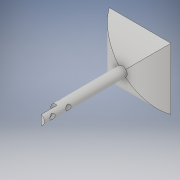
# Autodesk Inventor part: thumper-bumper-plunger
Saved by Autodesk Inventor 2017 (Build 210142000, 142)
## iProperties
Created: 2017-02-27
Part Number: thumper-bumper-plunger
Material: Generic
Document SubType Name: Modeling
Designer: John
Density: 1 g/cm^3
Appearance: Default
Author: John
Autodesk Inventor part; units mm, degrees
ref_plane "XZ Plane" through (0, 0, 0) normal (0, 1, 0) x (-1, 0, 0)
ref_plane "XY Plane" through (0, 0, 0) normal (0, 0, 1) x (1, 0, 0)
sketch "Sketch1" plane through (0, 0, 0) normal (0, 1, 0) x (-1, 0, 0)
  line L0 (0, 0) -> (3, 0)
  line L1 (3, 0) -> (3, 50)
  line L2 (3, 50) -> (0, 50)
  line L3 (0, 50) -> (0, 0)
  dimension "d0" = 3
  dimension "d1" = 50
  constraints: 8 end point, 2 parallel, 1 horizontal, 1 perpendicular
  measures "d0" distance of L2.end L1.end
  measures "d1" distance of L1.end L0.end
revolve "Revolution1" add sketch "Sketch1" angle 360 about axis through (0, 0, 50) along (0, 0, -1)
sketch "Sketch2" plane through (0, 0, 0) normal (0, 0, -1) x (-1, 0, 0)
  line L0 (-17.5, 17.5) -> (17.5, 17.5)
  line L1 (17.5, 17.5) -> (17.5, -17.5)
  line L2 (17.5, -17.5) -> (-17.5, -17.5)
  line L3 (-17.5, -17.5) -> (-17.5, 17.5)
  line L4 (-17.5, 17.5) -> (17.5, -17.5) construction
  line L5 (17.5, 17.5) -> (-17.5, -17.5) construction
  point P0 (0, 0)
  dimension "d6" = 35
  dimension "d7" = 35
  constraints: 12 end point, 2 midpoint, 2 parallel, 1 horizontal, 1 perpendicular
  measures "d6" distance of L1.end L2.end
  measures "d7" distance of L0.end L1.end
extrude "Extrusion1" add sketch "Sketch2" against normal blind 14
sketch "Sketch3" plane through (-17.5, 17.5, 0) normal (0, 1, 0) x (1, 0, 0)
  line L0 (35, 0) -> (35, -14) projected
  line L1 (0, 0) -> (35, 0)
  arc A0 (0, 0) -> (35, 0) centre (17.5, 9.6825) ccw
  point P0 (17.5, 0)
  dimension "d10" = 20
  dimension "d11" = 17.5
  constraints: 2 end point, 2 point on circle, 1 centre point, 1 perpendicular
  measures "d10" radius of A0
  measures "d11" distance from line of A0.centre L0
extrude "Extrusion2" cut sketch "Sketch3" against normal through all keep common part
sketch "Sketch4" plane through (17.5, -17.5, 0) normal (1, 0, 0) x (0, 0, -1)
  line L0 (0, 35) -> (0, 0) projected
  line L1 (0, 35) -> (0, 0)
  arc A0 (0, 35) -> (0, 0) centre (9.6825, 17.5) ccw
  point P0 (0, 17.5)
  dimension "d14" = 20
  constraints: 2 end point, 2 point on circle, 1 centre point, 1 collinear
  measures "d14" radius of A0
extrude "Extrusion3" cut sketch "Sketch4" against normal through all keep common part
sketch "Sketch5" plane through (17.5, 17.5, 0) normal (0, 0, -1) x (-1, 0, 0)
  line L0 (35, 0) -> (17.5, -17.5) projected
  circle A0 centre (17.5, -17.5) radius 2.75
  dimension "d17" = 5.5
  constraints: 1 centre point, 1 coincident
  measures "d17" diameter of A0
extrude "Extrusion4" add sketch "Sketch5" against normal blind 48
ref_plane "Work Plane1" through (0, 0, 0) normal (1, 0, 0) x (0, 1, 0)
sketch "Sketch6" plane through (0, 0, 48) normal (0, 0, 1) x (1, 0, 0)
  circle A0 centre (0, 0) radius 2.75 projected
  line L0 (0.8, -2.6311) -> (0.8, 2.6311)
  arc A1 (0.8, -2.6311) -> (0.8, 2.6311) centre (0, 0) ccw
  point P0 (0, 0)
  dimension "d28" = 0.8
  constraints: 4 point on circle, 2 end point, 1 centre point, 1 concentric, 1 vertical
  measures "d28" distance from line of point (0, 0) L0
extrude "Extrusion5" add sketch "Sketch6" along normal blind 9 contours A0 L0 picked at (0.979, 0.801)
sketch "Sketch7" plane through (0.8, -2.6311, 48) normal (-1, 0, 0) x (0, 0, 1)
  circle A0 centre (4.5, 2.75) radius 1.5
  line L0 (9, 5.2621) -> (9, 0) projected
  circle A1 centre (-4.5, 2.75) radius 1.5
  point P0 (-48, 2.6311)
  dimension "d23" = 3
  dimension "d24" = 4.5
  dimension "d31" = 3
  dimension "d32" = 9
  constraints: 2 centre point
  measures "d23" diameter of A0
  measures "d24" distance from line of L0 A0.centre
  measures "d31" diameter of A1
  measures "d32" distance of A1.centre A0.centre
extrude "Extrusion6" cut sketch "Sketch7" along normal through all both and the other way through all
equation "\"d7\" = d6"
body "Solid1"
